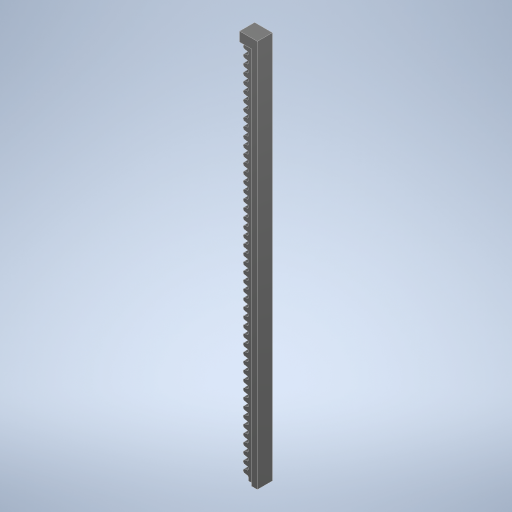
# Autodesk Inventor part: Hreben_Horizontal_cast
Saved by Autodesk Inventor 2024.2 (Build 282272000, 272)
## iProperties
Created: 2025-06-02
Part Number: Hreben_Horizontal_cast
Material: Termoplastická pryskyřice
Document SubType Name: Modeling
Designer: Elite
Density: 1.28 g/cm^3
Appearance: Hladká – černá
Mass: 4.51235 g
Surface Area: 29.4448 cm^2
Volume: 3.52528 cm^3
Author: Elite
Autodesk Inventor part; units mm, degrees
(part 1 of 2)
ref_plane "YZ Plane" through (0, 0, 0) normal (1, 0, 0) x (0, 1, 0)
ref_plane "XZ Plane" through (0, 0, 0) normal (0, 1, 0) x (-1, 0, 0)
ref_plane "XY Plane" through (0, 0, 0) normal (0, 0, 1) x (1, 0, 0)
sketch "Náčrt1" plane through (0, 0, 0) normal (0, 0, 1) x (1, 0, 0)
  line L0 (-2.539999, 6.35) -> (0, 6.35)
  line L1 (-2.539999, 6.35) -> (-3.809999, 5.08)
  line L2 (-3.809999, 5.08) -> (-5.079999, 5.08)
  line L3 (-5.079999, 5.08) -> (-5.079999, 1.27)
  line L4 (-5.079999, 1.27) -> (-3.809999, 1.27)
  line L5 (-3.809999, 1.27) -> (-2.539999, 0)
  line L6 (-2.539999, 0) -> (0, 0)
  line L7 (0, 0) -> (0, 6.35)
  constraints: 16 end point
extrude "Vysunutí1" add sketch "Náčrt1" against normal blind 160
sketch "Náčrt2" plane through (-3.809999, 5.08, 0) normal (0, 1, 0) x (1, 0, 0)
  line L0 (0, 0) -> (-1.27, 0)
  line L1 (0, 0) -> (0, 160)
  line L2 (-1.27, 160) -> (0, 160)
  line L3 (-1.27, 0) -> (-1.27, 160)
  arc A0 (-1.678461, 2.998415) -> (-1.27, 3.497336) centre (-1.778009, 3.496575) ccw
  arc A1 (-2.97646, 2.739034) -> (-3.389, 2.240304) centre (-2.881172, 2.240226) ccw
  arc A2 (-3.389, 1.845748) -> (-2.971901, 1.32351) centre (-2.881505, 1.82339) ccw
  line L4 (-2.990322, 1.327194) -> (-2.971901, 1.32351)
  arc A3 (-1.27, 0.566986) -> (-1.677758, 1.064456) centre (-1.777338, 0.566986) ccw
  line L5 (-1.27, 3.868884) -> (-1.27, 3.495814)
  line L6 (-1.27, 0) -> (-1.27, 160)
  line L7 (-2.971901, 1.32351) -> (-1.677758, 1.064456)
  line L8 (-3.389, 1.845748) -> (-3.389, 2.24059)
  line L9 (-2.97646, 2.739034) -> (-1.678461, 2.998415)
  line L10 (-1.27, 0.566986) -> (-1.27, 3.868884)
  arc A4 (-1.678461, 6.300312) -> (-1.27, 6.799234) centre (-1.778009, 6.798472) ccw
  arc A5 (-2.97646, 6.040931) -> (-3.389, 5.542202) centre (-2.881172, 5.542123) ccw
  arc A6 (-3.389, 5.147645) -> (-2.971901, 4.625407) centre (-2.881505, 5.125287) ccw
  line L11 (-2.990322, 4.629092) -> (-2.971901, 4.625407)
  arc A7 (-1.27, 3.868884) -> (-1.677758, 4.366353) centre (-1.777338, 3.868884) ccw
  line L12 (-1.27, 7.170781) -> (-1.27, 6.797711)
  line L13 (-2.971901, 4.625407) -> (-1.677758, 4.366353)
  line L14 (-3.389, 5.147645) -> (-3.389, 5.542488)
  line L15 (-2.97646, 6.040931) -> (-1.678461, 6.300312)
  line L16 (-1.27, 3.868884) -> (-1.27, 7.170781)
  arc A8 (-1.678461, 9.602209) -> (-1.27, 10.101131) centre (-1.778009, 10.10037) ccw
  arc A9 (-2.97646, 9.342828) -> (-3.389, 8.844099) centre (-2.881172, 8.844021) ccw
  arc A10 (-3.389, 8.449542) -> (-2.971901, 7.927305) centre (-2.881505, 8.427184) ccw
  line L17 (-2.990322, 7.930989) -> (-2.971901, 7.927305)
  arc A11 (-1.27, 7.170781) -> (-1.677758, 7.668251) centre (-1.777338, 7.170781) ccw
  line L18 (-1.27, 10.472678) -> (-1.27, 10.099608)
  line L19 (-2.971901, 7.927305) -> (-1.677758, 7.668251)
  line L20 (-3.389, 8.449542) -> (-3.389, 8.844385)
  line L21 (-2.97646, 9.342828) -> (-1.678461, 9.602209)
  line L22 (-1.27, 7.170781) -> (-1.27, 10.472678)
  arc A12 (-1.678461, 12.904106) -> (-1.27, 13.403028) centre (-1.778009, 13.402267) ccw
  arc A13 (-2.97646, 12.644726) -> (-3.389, 12.145996) centre (-2.881172, 12.145918) ccw
  arc A14 (-3.389, 11.751439) -> (-2.971901, 11.229202) centre (-2.881505, 11.729081) ccw
  line L23 (-2.990322, 11.232886) -> (-2.971901, 11.229202)
  arc A15 (-1.27, 10.472678) -> (-1.677758, 10.970148) centre (-1.777338, 10.472678) ccw
  line L24 (-1.27, 13.774575) -> (-1.27, 13.401505)
  line L25 (-2.971901, 11.229202) -> (-1.677758, 10.970148)
  line L26 (-3.389, 11.751439) -> (-3.389, 12.146282)
  line L27 (-2.97646, 12.644726) -> (-1.678461, 12.904106)
  line L28 (-1.27, 10.472678) -> (-1.27, 13.774575)
  arc A16 (-1.678461, 16.206003) -> (-1.27, 16.704925) centre (-1.778009, 16.704164) ccw
  arc A17 (-2.97646, 15.946623) -> (-3.389, 15.447893) centre (-2.881172, 15.447815) ccw
  arc A18 (-3.389, 15.053337) -> (-2.971901, 14.531099) centre (-2.881505, 15.030979) ccw
  line L29 (-2.990322, 14.534783) -> (-2.971901, 14.531099)
  arc A19 (-1.27, 13.774575) -> (-1.677758, 14.272045) centre (-1.777338, 13.774575) ccw
  line L30 (-1.27, 17.076472) -> (-1.27, 16.703403)
  line L31 (-2.971901, 14.531099) -> (-1.677758, 14.272045)
  line L32 (-3.389, 15.053337) -> (-3.389, 15.448179)
  line L33 (-2.97646, 15.946623) -> (-1.678461, 16.206003)
  line L34 (-1.27, 13.774575) -> (-1.27, 17.076472)
  arc A20 (-1.678461, 19.507901) -> (-1.27, 20.006822) centre (-1.778009, 20.006061) ccw
  arc A21 (-2.97646, 19.24852) -> (-3.389, 18.74979) centre (-2.881172, 18.749712) ccw
  arc A22 (-3.389, 18.355234) -> (-2.971901, 17.832996) centre (-2.881505, 18.332876) ccw
  line L35 (-2.990322, 17.83668) -> (-2.971901, 17.832996)
  arc A23 (-1.27, 17.076472) -> (-1.677758, 17.573942) centre (-1.777338, 17.076472) ccw
  line L36 (-1.27, 20.37837) -> (-1.27, 20.0053)
  line L37 (-2.971901, 17.832996) -> (-1.677758, 17.573942)
  line L38 (-3.389, 18.355234) -> (-3.389, 18.750076)
  line L39 (-2.97646, 19.24852) -> (-1.678461, 19.507901)
  line L40 (-1.27, 17.076472) -> (-1.27, 20.37837)
  arc A24 (-1.678461, 22.809798) -> (-1.27, 23.30872) centre (-1.778009, 23.307958) ccw
  arc A25 (-2.97646, 22.550417) -> (-3.389, 22.051688) centre (-2.881172, 22.051609) ccw
  arc A26 (-3.389, 21.657131) -> (-2.971901, 21.134893) centre (-2.881505, 21.634773) ccw
  line L41 (-2.990322, 21.138578) -> (-2.971901, 21.134893)
  arc A27 (-1.27, 20.37837) -> (-1.677758, 20.875839) centre (-1.777338, 20.37837) ccw
  line L42 (-1.27, 23.680267) -> (-1.27, 23.307197)
  line L43 (-2.971901, 21.134893) -> (-1.677758, 20.875839)
  line L44 (-3.389, 21.657131) -> (-3.389, 22.051974)
  line L45 (-2.97646, 22.550417) -> (-1.678461, 22.809798)
  line L46 (-1.27, 20.37837) -> (-1.27, 23.680267)
  arc A28 (-1.678461, 26.111695) -> (-1.27, 26.610617) centre (-1.778009, 26.609856) ccw
  arc A29 (-2.97646, 25.852314) -> (-3.389, 25.353585) centre (-2.881172, 25.353507) ccw
  arc A30 (-3.389, 24.959028) -> (-2.971901, 24.436791) centre (-2.881505, 24.93667) ccw
  line L47 (-2.990322, 24.440475) -> (-2.971901, 24.436791)
  arc A31 (-1.27, 23.680267) -> (-1.677758, 24.177737) centre (-1.777338, 23.680267) ccw
  line L48 (-1.27, 26.982164) -> (-1.27, 26.609094)
  line L49 (-2.971901, 24.436791) -> (-1.677758, 24.177737)
  line L50 (-3.389, 24.959028) -> (-3.389, 25.353871)
  line L51 (-2.97646, 25.852314) -> (-1.678461, 26.111695)
  line L52 (-1.27, 23.680267) -> (-1.27, 26.982164)
  line L53 (-2.971901, 27.738688) -> (-1.677758, 27.479634)
  line L54 (-2.97646, 29.154212) -> (-1.678461, 29.413592)
  line L55 (-2.990322, 27.742372) -> (-2.971901, 27.738688)
  arc A32 (-2.97646, 29.154212) -> (-3.389, 28.655482) centre (-2.881172, 28.655404) ccw
  line L56 (-3.389, 28.260925) -> (-3.389, 28.655768)
  arc A33 (-3.389, 28.260925) -> (-2.971901, 27.738688) centre (-2.881505, 28.238567) ccw
  arc A34 (-1.27, 26.982164) -> (-1.677758, 27.479634) centre (-1.777338, 26.982164) ccw
  arc A35 (-1.678461, 29.413592) -> (-1.27, 29.912514) centre (-1.778009, 29.911753) ccw
  line L57 (-1.27, 30.284061) -> (-1.27, 29.910991)
  line L58 (-1.27, 26.982164) -> (-1.27, 30.284061)
  line L59 (-2.971901, 31.040585) -> (-1.677758, 30.781531)
  line L60 (-2.97646, 32.456109) -> (-1.678461, 32.715489)
  line L61 (-2.990322, 31.044269) -> (-2.971901, 31.040585)
  arc A36 (-2.97646, 32.456109) -> (-3.389, 31.957379) centre (-2.881172, 31.957301) ccw
  line L62 (-3.389, 31.562823) -> (-3.389, 31.957665)
  arc A37 (-3.389, 31.562823) -> (-2.971901, 31.040585) centre (-2.881505, 31.540465) ccw
  arc A38 (-1.27, 30.284061) -> (-1.677758, 30.781531) centre (-1.777338, 30.284061) ccw
  arc A39 (-1.678461, 32.715489) -> (-1.27, 33.214411) centre (-1.778009, 33.21365) ccw
  line L63 (-1.27, 33.585958) -> (-1.27, 33.212889)
  line L64 (-1.27, 30.284061) -> (-1.27, 33.585958)
  line L65 (-2.971901, 34.342482) -> (-1.677758, 34.083428)
  line L66 (-2.97646, 35.758006) -> (-1.678461, 36.017387)
  line L67 (-2.990322, 34.346166) -> (-2.971901, 34.342482)
  arc A40 (-2.97646, 35.758006) -> (-3.389, 35.259276) centre (-2.881172, 35.259198) ccw
  line L68 (-3.389, 34.86472) -> (-3.389, 35.259562)
  arc A41 (-3.389, 34.86472) -> (-2.971901, 34.342482) centre (-2.881505, 34.842362) ccw
  arc A42 (-1.27, 33.585958) -> (-1.677758, 34.083428) centre (-1.777338, 33.585958) ccw
  arc A43 (-1.678461, 36.017387) -> (-1.27, 36.516308) centre (-1.778009, 36.515547) ccw
  line L69 (-1.27, 36.887856) -> (-1.27, 36.514786)
  line L70 (-1.27, 33.585958) -> (-1.27, 36.887856)
  line L71 (-2.971901, 37.644379) -> (-1.677758, 37.385325)
  line L72 (-2.97646, 39.059903) -> (-1.678461, 39.319284)
  line L73 (-2.990322, 37.648064) -> (-2.971901, 37.644379)
  arc A44 (-2.97646, 39.059903) -> (-3.389, 38.561174) centre (-2.881172, 38.561095) ccw
  line L74 (-3.389, 38.166617) -> (-3.389, 38.56146)
  arc A45 (-3.389, 38.166617) -> (-2.971901, 37.644379) centre (-2.881505, 38.144259) ccw
  arc A46 (-1.27, 36.887856) -> (-1.677758, 37.385325) centre (-1.777338, 36.887856) ccw
  arc A47 (-1.678461, 39.319284) -> (-1.27, 39.818206) centre (-1.778009, 39.817444) ccw
  line L75 (-1.27, 40.189753) -> (-1.27, 39.816683)
  line L76 (-1.27, 36.887856) -> (-1.27, 40.189753)
  line L77 (-2.971901, 40.946276) -> (-1.677758, 40.687223)
  line L78 (-2.97646, 42.3618) -> (-1.678461, 42.621181)
  line L79 (-2.990322, 40.949961) -> (-2.971901, 40.946276)
  arc A48 (-2.97646, 42.3618) -> (-3.389, 41.863071) centre (-2.881172, 41.862993) ccw
  line L80 (-3.389, 41.468514) -> (-3.389, 41.863357)
  arc A49 (-3.389, 41.468514) -> (-2.971901, 40.946276) centre (-2.881505, 41.446156) ccw
  arc A50 (-1.27, 40.189753) -> (-1.677758, 40.687223) centre (-1.777338, 40.189753) ccw
  arc A51 (-1.678461, 42.621181) -> (-1.27, 43.120103) centre (-1.778009, 43.119342) ccw
  line L81 (-1.27, 43.49165) -> (-1.27, 43.11858)
  line L82 (-1.27, 40.189753) -> (-1.27, 43.49165)
  line L83 (-2.971901, 44.248174) -> (-1.677758, 43.98912)
  line L84 (-2.97646, 45.663698) -> (-1.678461, 45.923078)
  line L85 (-2.990322, 44.251858) -> (-2.971901, 44.248174)
  arc A52 (-2.97646, 45.663698) -> (-3.389, 45.164968) centre (-2.881172, 45.16489) ccw
  line L86 (-3.389, 44.770411) -> (-3.389, 45.165254)
  arc A53 (-3.389, 44.770411) -> (-2.971901, 44.248174) centre (-2.881505, 44.748053) ccw
  arc A54 (-1.27, 43.49165) -> (-1.677758, 43.98912) centre (-1.777338, 43.49165) ccw
  arc A55 (-1.678461, 45.923078) -> (-1.27, 46.422) centre (-1.778009, 46.421239) ccw
  line L87 (-1.27, 46.793547) -> (-1.27, 46.420477)
  line L88 (-1.27, 43.49165) -> (-1.27, 46.793547)
  arc A56 (-1.678461, 49.224975) -> (-1.27, 49.723897) centre (-1.778009, 49.723136) ccw
  arc A57 (-2.97646, 48.965595) -> (-3.389, 48.466865) centre (-2.881172, 48.466787) ccw
  arc A58 (-3.389, 48.072309) -> (-2.971901, 47.550071) centre (-2.881505, 48.049951) ccw
  line L89 (-2.990322, 47.553755) -> (-2.971901, 47.550071)
  arc A59 (-1.27, 46.793547) -> (-1.677758, 47.291017) centre (-1.777338, 46.793547) ccw
  line L90 (-1.27, 50.095444) -> (-1.27, 49.722375)
  line L91 (-2.971901, 47.550071) -> (-1.677758, 47.291017)
  line L92 (-3.389, 48.072309) -> (-3.389, 48.467151)
  line L93 (-2.97646, 48.965595) -> (-1.678461, 49.224975)
  line L94 (-1.27, 46.793547) -> (-1.27, 50.095444)
  line L95 (-2.971901, 50.851968) -> (-1.677758, 50.592914)
  line L96 (-2.97646, 52.267492) -> (-1.678461, 52.526873)
  line L97 (-2.990322, 50.855652) -> (-2.971901, 50.851968)
  arc A60 (-2.97646, 52.267492) -> (-3.389, 51.768762) centre (-2.881172, 51.768684) ccw
  line L98 (-3.389, 51.374206) -> (-3.389, 51.769048)
  arc A61 (-3.389, 51.374206) -> (-2.971901, 50.851968) centre (-2.881505, 51.351848) ccw
  arc A62 (-1.27, 50.095444) -> (-1.677758, 50.592914) centre (-1.777338, 50.095444) ccw
  arc A63 (-1.678461, 52.526873) -> (-1.27, 53.025794) centre (-1.778009, 53.025033) ccw
  line L99 (-1.27, 53.397342) -> (-1.27, 53.024272)
  line L100 (-1.27, 50.095444) -> (-1.27, 53.397342)
  line L101 (-2.971901, 54.153865) -> (-1.677758, 53.894811)
  line L102 (-2.97646, 55.569389) -> (-1.678461, 55.82877)
  line L103 (-2.990322, 54.15755) -> (-2.971901, 54.153865)
  arc A64 (-2.97646, 55.569389) -> (-3.389, 55.07066) centre (-2.881172, 55.070581) ccw
  line L104 (-3.389, 54.676103) -> (-3.389, 55.070946)
  arc A65 (-3.389, 54.676103) -> (-2.971901, 54.153865) centre (-2.881505, 54.653745) ccw
  arc A66 (-1.27, 53.397342) -> (-1.677758, 53.894811) centre (-1.777338, 53.397342) ccw
  arc A67 (-1.678461, 55.82877) -> (-1.27, 56.327692) centre (-1.778009, 56.32693) ccw
  line L105 (-1.27, 56.699239) -> (-1.27, 56.326169)
  line L106 (-1.27, 53.397342) -> (-1.27, 56.699239)
  line L107 (-2.971901, 57.455762) -> (-1.677758, 57.196709)
  line L108 (-2.97646, 58.871286) -> (-1.678461, 59.130667)
  line L109 (-2.990322, 57.459447) -> (-2.971901, 57.455762)
  arc A68 (-2.97646, 58.871286) -> (-3.389, 58.372557) centre (-2.881172, 58.372479) ccw
  line L110 (-3.389, 57.978) -> (-3.389, 58.372843)
  arc A69 (-3.389, 57.978) -> (-2.971901, 57.455762) centre (-2.881505, 57.955642) ccw
  arc A70 (-1.27, 56.699239) -> (-1.677758, 57.196709) centre (-1.777338, 56.699239) ccw
  arc A71 (-1.678461, 59.130667) -> (-1.27, 59.629589) centre (-1.778009, 59.628828) ccw
  line L111 (-1.27, 60.001136) -> (-1.27, 59.628066)
  line L112 (-1.27, 56.699239) -> (-1.27, 60.001136)
  line L113 (-2.971901, 60.75766) -> (-1.677758, 60.498606)
  line L114 (-2.97646, 62.173184) -> (-1.678461, 62.432564)
  line L115 (-2.990322, 60.761344) -> (-2.971901, 60.75766)
  arc A72 (-2.97646, 62.173184) -> (-3.389, 61.674454) centre (-2.881172, 61.674376) ccw
  line L116 (-3.389, 61.279897) -> (-3.389, 61.67474)
  arc A73 (-3.389, 61.279897) -> (-2.971901, 60.75766) centre (-2.881505, 61.257539) ccw
  arc A74 (-1.27, 60.001136) -> (-1.677758, 60.498606) centre (-1.777338, 60.001136) ccw
  arc A75 (-1.678461, 62.432564) -> (-1.27, 62.931486) centre (-1.778009, 62.930725) ccw
  line L117 (-1.27, 63.303033) -> (-1.27, 62.929963)
  line L118 (-1.27, 60.001136) -> (-1.27, 63.303033)
  line L119 (-2.971901, 64.059557) -> (-1.677758, 63.800503)
  line L120 (-2.97646, 65.475081) -> (-1.678461, 65.734461)
  line L121 (-2.990322, 64.063241) -> (-2.971901, 64.059557)
  arc A76 (-2.97646, 65.475081) -> (-3.389, 64.976351) centre (-2.881172, 64.976273) ccw
  line L122 (-3.389, 64.581795) -> (-3.389, 64.976637)
  arc A77 (-3.389, 64.581795) -> (-2.971901, 64.059557) centre (-2.881505, 64.559437) ccw
  arc A78 (-1.27, 63.303033) -> (-1.677758, 63.800503) centre (-1.777338, 63.303033) ccw
  arc A79 (-1.678461, 65.734461) -> (-1.27, 66.233383) centre (-1.778009, 66.232622) ccw
  line L123 (-1.27, 66.60493) -> (-1.27, 66.231861)
  line L124 (-1.27, 63.303033) -> (-1.27, 66.60493)
  line L125 (-2.971901, 67.361454) -> (-1.677758, 67.1024)
  line L126 (-2.97646, 68.776978) -> (-1.678461, 69.036358)
  line L127 (-2.990322, 67.365138) -> (-2.971901, 67.361454)
  arc A80 (-2.97646, 68.776978) -> (-3.389, 68.278248) centre (-2.881172, 68.27817) ccw
  line L128 (-3.389, 67.883692) -> (-3.389, 68.278534)
  arc A81 (-3.389, 67.883692) -> (-2.971901, 67.361454) centre (-2.881505, 67.861334) ccw
  arc A82 (-1.27, 66.60493) -> (-1.677758, 67.1024) centre (-1.777338, 66.60493) ccw
  arc A83 (-1.678461, 69.036358) -> (-1.27, 69.53528) centre (-1.778009, 69.534519) ccw
  line L129 (-1.27, 69.906828) -> (-1.27, 69.533758)
  line L130 (-1.27, 66.60493) -> (-1.27, 69.906828)
  arc A84 (-1.678461, 72.338256) -> (-1.27, 72.837178) centre (-1.778009, 72.836416) ccw
  arc A85 (-2.97646, 72.078875) -> (-3.389, 71.580145) centre (-2.881172, 71.580067) ccw
  arc A86 (-3.389, 71.185589) -> (-2.971901, 70.663351) centre (-2.881505, 71.163231) ccw
  line L131 (-2.990322, 70.667035) -> (-2.971901, 70.663351)
  arc A87 (-1.27, 69.906828) -> (-1.677758, 70.404297) centre (-1.777338, 69.906828) ccw
  line L132 (-1.27, 73.208725) -> (-1.27, 72.835655)
  line L133 (-2.971901, 70.663351) -> (-1.677758, 70.404297)
  line L134 (-3.389, 71.185589) -> (-3.389, 71.580432)
  line L135 (-2.97646, 72.078875) -> (-1.678461, 72.338256)
  line L136 (-1.27, 69.906828) -> (-1.27, 73.208725)
  line L137 (-2.971901, 73.965248) -> (-1.677758, 73.706195)
  line L138 (-2.97646, 75.380772) -> (-1.678461, 75.640153)
  line L139 (-2.990322, 73.968933) -> (-2.971901, 73.965248)
  arc A88 (-2.97646, 75.380772) -> (-3.389, 74.882043) centre (-2.881172, 74.881965) ccw
  line L140 (-3.389, 74.487486) -> (-3.389, 74.882329)
  arc A89 (-3.389, 74.487486) -> (-2.971901, 73.965248) centre (-2.881505, 74.465128) ccw
  arc A90 (-1.27, 73.208725) -> (-1.677758, 73.706195) centre (-1.777338, 73.208725) ccw
  arc A91 (-1.678461, 75.640153) -> (-1.27, 76.139075) centre (-1.778009, 76.138314) ccw
  line L141 (-1.27, 76.510622) -> (-1.27, 76.137552)
  line L142 (-1.27, 73.208725) -> (-1.27, 76.510622)
  line L143 (-2.971901, 77.267146) -> (-1.677758, 77.008092)
  line L144 (-2.97646, 78.68267) -> (-1.678461, 78.94205)
  line L145 (-2.990322, 77.27083) -> (-2.971901, 77.267146)
  arc A92 (-2.97646, 78.68267) -> (-3.389, 78.18394) centre (-2.881172, 78.183862) ccw
  line L146 (-3.389, 77.789383) -> (-3.389, 78.184226)
  arc A93 (-3.389, 77.789383) -> (-2.971901, 77.267146) centre (-2.881505, 77.767025) ccw
  arc A94 (-1.27, 76.510622) -> (-1.677758, 77.008092) centre (-1.777338, 76.510622) ccw
  arc A95 (-1.678461, 78.94205) -> (-1.27, 79.440972) centre (-1.778009, 79.440211) ccw
  line L147 (-1.27, 79.812519) -> (-1.27, 79.439449)
  line L148 (-1.27, 76.510622) -> (-1.27, 79.812519)
  line L149 (-2.971901, 80.569043) -> (-1.677758, 80.309989)
  line L150 (-2.97646, 81.984567) -> (-1.678461, 82.243947)
  line L151 (-2.990322, 80.572727) -> (-2.971901, 80.569043)
  arc A96 (-2.97646, 81.984567) -> (-3.389, 81.485837) centre (-2.881172, 81.485759) ccw
  line L152 (-3.389, 81.091281) -> (-3.389, 81.486123)
  arc A97 (-3.389, 81.091281) -> (-2.971901, 80.569043) centre (-2.881505, 81.068923) ccw
  arc A98 (-1.27, 79.812519) -> (-1.677758, 80.309989) centre (-1.777338, 79.812519) ccw
  arc A99 (-1.678461, 82.243947) -> (-1.27, 82.742869) centre (-1.778009, 82.742108) ccw
  line L153 (-1.27, 83.114416) -> (-1.27, 82.741347)
  line L154 (-1.27, 79.812519) -> (-1.27, 83.114416)
  line L155 (-2.971901, 83.87094) -> (-1.677758, 83.611886)
  line L156 (-2.97646, 85.286464) -> (-1.678461, 85.545844)
  line L157 (-2.990322, 83.874624) -> (-2.971901, 83.87094)
  arc A100 (-2.97646, 85.286464) -> (-3.389, 84.787734) centre (-2.881172, 84.787656) ccw
  line L158 (-3.389, 84.393178) -> (-3.389, 84.78802)
  arc A101 (-3.389, 84.393178) -> (-2.971901, 83.87094) centre (-2.881505, 84.37082) ccw
  arc A102 (-1.27, 83.114416) -> (-1.677758, 83.611886) centre (-1.777338, 83.114416) ccw
  arc A103 (-1.678461, 85.545844) -> (-1.27, 86.044766) centre (-1.778009, 86.044005) ccw
  line L159 (-1.27, 86.416314) -> (-1.27, 86.043244)
  line L160 (-1.27, 83.114416) -> (-1.27, 86.416314)
  line L161 (-2.971901, 87.172837) -> (-1.677758, 86.913783)
  line L162 (-2.97646, 88.588361) -> (-1.678461, 88.847742)
  line L163 (-2.990322, 87.176521) -> (-2.971901, 87.172837)
  arc A104 (-2.97646, 88.588361) -> (-3.389, 88.089631) centre (-2.881172, 88.089553) ccw
  line L164 (-3.389, 87.695075) -> (-3.389, 88.089918)
  arc A105 (-3.389, 87.695075) -> (-2.971901, 87.172837) centre (-2.881505, 87.672717) ccw
  arc A106 (-1.27, 86.416314) -> (-1.677758, 86.913783) centre (-1.777338, 86.416314) ccw
  arc A107 (-1.678461, 88.847742) -> (-1.27, 89.346664) centre (-1.778009, 89.345902) ccw
  line L165 (-1.27, 89.718211) -> (-1.27, 89.345141)
  line L166 (-1.27, 86.416314) -> (-1.27, 89.718211)
  arc A108 (-1.27, 89.718211) -> (-1.677758, 90.215681) centre (-1.777338, 89.718211) ccw
  line L167 (-2.971901, 90.474734) -> (-1.677758, 90.215681)
  line L168 (-2.990322, 90.478419) -> (-2.971901, 90.474734)
  arc A109 (-3.389, 90.996972) -> (-2.971901, 90.474734) centre (-2.881505, 90.974614) ccw
  arc A110 (-2.97646, 91.890258) -> (-3.389, 91.391529) centre (-2.881172, 91.391451) ccw
  line L169 (-2.97646, 91.890258) -> (-1.678461, 92.149639)
  line L170 (-1.27, 89.718211) -> (-1.27, 93.020108)
  arc A111 (-1.678461, 92.149639) -> (-1.27, 92.648561) centre (-1.778009, 92.647799) ccw
  line L171 (-1.27, 93.020108) -> (-1.27, 92.647038)
  line L172 (-3.389, 90.996972) -> (-3.389, 91.391815)
  arc A112 (-1.27, 93.020108) -> (-1.677758, 93.517578) centre (-1.777338, 93.020108) ccw
  line L173 (-2.971901, 93.776632) -> (-1.677758, 93.517578)
  line L174 (-2.990322, 93.780316) -> (-2.971901, 93.776632)
  arc A113 (-3.389, 94.298869) -> (-2.971901, 93.776632) centre (-2.881505, 94.276511) ccw
  line L175 (-3.389, 94.298869) -> (-3.389, 94.693712)
  arc A114 (-2.97646, 95.192156) -> (-3.389, 94.693426) centre (-2.881172, 94.693348) ccw
  line L176 (-1.27, 93.020108) -> (-1.27, 96.322005)
  line L177 (-2.97646, 95.192156) -> (-1.678461, 95.451536)
  arc A115 (-1.678461, 95.451536) -> (-1.27, 95.950458) centre (-1.778009, 95.949697) ccw
  line L178 (-1.27, 96.322005) -> (-1.27, 95.948935)
  arc A116 (-1.678461, 98.753433) -> (-1.27, 99.252355) centre (-1.778009, 99.251594) ccw
  arc A117 (-1.27, 99.623902) -> (-1.677758, 100.121372) centre (-1.777338, 99.623902) ccw
  line L179 (-1.27, 99.623902) -> (-1.27, 99.250833)
  arc A118 (-2.97646, 98.494053) -> (-3.389, 97.995323) centre (-2.881172, 97.995245) ccw
  line L180 (-2.990322, 97.082213) -> (-2.971901, 97.078529)
  arc A119 (-3.389, 97.600767) -> (-2.971901, 97.078529) centre (-2.881505, 97.578409) ccw
  line L181 (-2.971901, 100.380426) -> (-1.677758, 100.121372)
  line L182 (-2.990322, 100.38411) -> (-2.971901, 100.380426)
  arc A120 (-3.389, 100.902664) -> (-2.971901, 100.380426) centre (-2.881505, 100.880306) ccw
  line L183 (-3.389, 100.902664) -> (-3.389, 101.297506)
  arc A121 (-2.97646, 101.79595) -> (-3.389, 101.29722) centre (-2.881172, 101.297142) ccw
  line L184 (-2.97646, 101.79595) -> (-1.678461, 102.05533)
  line L185 (-1.27, 99.623902) -> (-1.27, 102.925799)
  arc A122 (-1.678461, 102.05533) -> (-1.27, 102.554252) centre (-1.778009, 102.553491) ccw
  line L186 (-1.27, 102.925799) -> (-1.27, 102.55273)
  arc A123 (-1.27, 96.322005) -> (-1.677758, 96.819475) centre (-1.777338, 96.322005) ccw
  line L187 (-2.971901, 97.078529) -> (-1.677758, 96.819475)
  line L188 (-2.97646, 98.494053) -> (-1.678461, 98.753433)
  line L189 (-3.389, 97.600767) -> (-3.389, 97.995609)
  line L190 (-1.27, 96.322005) -> (-1.27, 99.623902)
  arc A124 (-1.27, 102.925799) -> (-1.677758, 103.423269) centre (-1.777338, 102.925799) ccw
  line L191 (-2.971901, 103.682323) -> (-1.677758, 103.423269)
  line L192 (-2.990322, 103.686007) -> (-2.971901, 103.682323)
  arc A125 (-3.389, 104.204561) -> (-2.971901, 103.682323) centre (-2.881505, 104.182203) ccw
  line L193 (-3.389, 104.204561) -> (-3.389, 104.599404)
  arc A126 (-2.97646, 105.097847) -> (-3.389, 104.599117) centre (-2.881172, 104.599039) ccw
  line L194 (-2.97646, 105.097847) -> (-1.678461, 105.357228)
  line L195 (-1.27, 102.925799) -> (-1.27, 106.227697)
  arc A127 (-1.678461, 105.357228) -> (-1.27, 105.85615) centre (-1.778009, 105.855388) ccw
  line L196 (-1.27, 106.227697) -> (-1.27, 105.854627)
  arc A128 (-1.27, 106.227697) -> (-1.677758, 106.725166) centre (-1.777338, 106.227697) ccw
  line L197 (-2.971901, 106.98422) -> (-1.677758, 106.725166)
  line L198 (-2.990322, 106.987905) -> (-2.971901, 106.98422)
  arc A129 (-3.389, 107.506458) -> (-2.971901, 106.98422) centre (-2.881505, 107.4841) ccw
  line L199 (-3.389, 107.506458) -> (-3.389, 107.901301)
  arc A130 (-2.97646, 108.399744) -> (-3.389, 107.901015) centre (-2.881172, 107.900937) ccw
  line L200 (-2.97646, 108.399744) -> (-1.678461, 108.659125)
  line L201 (-1.27, 106.227697) -> (-1.27, 109.529594)
  arc A131 (-1.678461, 108.659125) -> (-1.27, 109.158047) centre (-1.778009, 109.157285) ccw
  line L202 (-1.27, 109.529594) -> (-1.27, 109.156524)
  arc A132 (-1.27, 109.529594) -> (-1.677758, 110.027064) centre (-1.777338, 109.529594) ccw
  line L203 (-2.971901, 110.286118) -> (-1.677758, 110.027064)
  line L204 (-2.990322, 110.289802) -> (-2.971901, 110.286118)
  line L205 (-3.389, 110.808355) -> (-3.389, 111.203198)
  arc A133 (-2.97646, 111.701641) -> (-3.389, 111.202912) centre (-2.881172, 111.202834) ccw
  line L206 (-2.97646, 111.701641) -> (-1.678461, 111.961022)
  arc A134 (-1.678461, 111.961022) -> (-1.27, 112.459944) centre (-1.778009, 112.459183) ccw
  line L207 (-1.27, 109.529594) -> (-1.27, 112.831491)
  line L208 (-1.27, 112.831491) -> (-1.27, 112.458421)
  arc A135 (-3.389, 110.808355) -> (-2.971901, 110.286118) centre (-2.881505, 110.785997) ccw
  arc A136 (-1.27, 112.831491) -> (-1.677758, 113.328961) centre (-1.777338, 112.831491) ccw
  line L209 (-2.971901, 113.588015) -> (-1.677758, 113.328961)
  line L210 (-2.990322, 113.591699) -> (-2.971901, 113.588015)
  arc A137 (-3.389, 114.110253) -> (-2.971901, 113.588015) centre (-2.881505, 114.087895) ccw
  arc A138 (-2.97646, 115.003539) -> (-3.389, 114.504809) centre (-2.881172, 114.504731) ccw
  line L211 (-2.97646, 115.003539) -> (-1.678461, 115.262919)
  line L212 (-1.27, 112.831491) -> (-1.27, 116.133388)
  arc A139 (-1.678461, 115.262919) -> (-1.27, 115.761841) centre (-1.778009, 115.76108) ccw
  line L213 (-1.27, 116.133388) -> (-1.27, 115.760319)
  line L214 (-3.389, 114.110253) -> (-3.389, 114.505095)
  arc A140 (-1.27, 116.133388) -> (-1.677758, 116.630858) centre (-1.777338, 116.133388) ccw
  line L215 (-2.971901, 116.889912) -> (-1.677758, 116.630858)
  line L216 (-2.990322, 116.893596) -> (-2.971901, 116.889912)
  arc A141 (-3.389, 117.41215) -> (-2.971901, 116.889912) centre (-2.881505, 117.389792) ccw
  line L217 (-3.389, 117.41215) -> (-3.389, 117.806992)
  arc A142 (-2.97646, 118.305436) -> (-3.389, 117.806706) centre (-2.881172, 117.806628) ccw
  line L218 (-1.27, 116.133388) -> (-1.27, 119.435285)
  line L219 (-2.97646, 118.305436) -> (-1.678461, 118.564816)
  arc A143 (-1.678461, 118.564816) -> (-1.27, 119.063738) centre (-1.778009, 119.062977) ccw
  line L220 (-1.27, 119.435285) -> (-1.27, 119.062216)
  arc A144 (-1.678461, 121.866714) -> (-1.27, 122.365636) centre (-1.778009, 122.364874) ccw
  arc A145 (-1.27, 122.737183) -> (-1.677758, 123.234652) centre (-1.777338, 122.737183) ccw
  line L221 (-1.27, 122.737183) -> (-1.27, 122.364113)
  arc A146 (-2.97646, 121.607333) -> (-3.389, 121.108603) centre (-2.881172, 121.108525) ccw
  line L222 (-2.990322, 120.195493) -> (-2.971901, 120.191809)
  arc A147 (-3.389, 120.714047) -> (-2.971901, 120.191809) centre (-2.881505, 120.691689) ccw
  line L223 (-2.971901, 123.493706) -> (-1.677758, 123.234652)
  line L224 (-2.990322, 123.497391) -> (-2.971901, 123.493706)
  arc A148 (-3.389, 124.015944) -> (-2.971901, 123.493706) centre (-2.881505, 123.993586) ccw
  line L225 (-3.389, 124.015944) -> (-3.389, 124.410787)
  arc A149 (-2.97646, 124.90923) -> (-3.389, 124.410501) centre (-2.881172, 124.410423) ccw
  line L226 (-2.97646, 124.90923) -> (-1.678461, 125.168611)
  line L227 (-1.27, 122.737183) -> (-1.27, 126.03908)
  arc A150 (-1.678461, 125.168611) -> (-1.27, 125.667533) centre (-1.778009, 125.666771) ccw
  line L228 (-1.27, 126.03908) -> (-1.27, 125.66601)
  arc A151 (-1.27, 119.435285) -> (-1.677758, 119.932755) centre (-1.777338, 119.435285) ccw
  line L229 (-2.971901, 120.191809) -> (-1.677758, 119.932755)
  line L230 (-2.97646, 121.607333) -> (-1.678461, 121.866714)
  line L231 (-3.389, 120.714047) -> (-3.389, 121.10889)
  line L232 (-1.27, 119.435285) -> (-1.27, 122.737183)
  arc A152 (-1.27, 126.03908) -> (-1.677758, 126.53655) centre (-1.777338, 126.03908) ccw
  line L233 (-2.971901, 126.795604) -> (-1.677758, 126.53655)
  line L234 (-2.990322, 126.799288) -> (-2.971901, 126.795604)
  arc A153 (-3.389, 127.317841) -> (-2.971901, 126.795604) centre (-2.881505, 127.295483) ccw
  line L235 (-3.389, 127.317841) -> (-3.389, 127.712684)
  arc A154 (-2.97646, 128.211127) -> (-3.389, 127.712398) centre (-2.881172, 127.71232) ccw
  line L236 (-2.97646, 128.211127) -> (-1.678461, 128.470508)
  line L237 (-1.27, 126.03908) -> (-1.27, 129.340977)
  arc A155 (-1.678461, 128.470508) -> (-1.27, 128.96943) centre (-1.778009, 128.968669) ccw
  line L238 (-1.27, 129.340977) -> (-1.27, 128.967907)
  arc A156 (-1.27, 129.340977) -> (-1.677758, 129.838447) centre (-1.777338, 129.340977) ccw
  line L239 (-2.971901, 130.097501) -> (-1.677758, 129.838447)
  line L240 (-2.990322, 130.101185) -> (-2.971901, 130.097501)
  arc A157 (-3.389, 130.619739) -> (-2.971901, 130.097501) centre (-2.881505, 130.59738) ccw
  line L241 (-3.389, 130.619739) -> (-3.389, 131.014581)
  arc A158 (-2.97646, 131.513025) -> (-3.389, 131.014295) centre (-2.881172, 131.014217) ccw
  line L242 (-2.97646, 131.513025) -> (-1.678461, 131.772405)
  line L243 (-1.27, 129.340977) -> (-1.27, 132.642874)
  arc A159 (-1.678461, 131.772405) -> (-1.27, 132.271327) centre (-1.778009, 132.270566) ccw
  line L244 (-1.27, 132.642874) -> (-1.27, 132.269805)
  arc A160 (-1.27, 132.642874) -> (-1.677758, 133.140344) centre (-1.777338, 132.642874) ccw
  line L245 (-2.971901, 133.399398) -> (-1.677758, 133.140344)
  line L246 (-2.990322, 133.403082) -> (-2.971901, 133.399398)
  line L247 (-3.389, 133.921636) -> (-3.389, 134.316478)
  arc A161 (-2.97646, 134.814922) -> (-3.389, 134.316192) centre (-2.881172, 134.316114) ccw
  line L248 (-2.97646, 134.814922) -> (-1.678461, 135.074302)
  arc A162 (-1.678461, 135.074302) -> (-1.27, 135.573224) centre (-1.778009, 135.572463) ccw
  line L249 (-1.27, 132.642874) -> (-1.27, 135.944771)
  line L250 (-1.27, 135.944771) -> (-1.27, 135.571702)
  arc A163 (-3.389, 133.921636) -> (-2.971901, 133.399398) centre (-2.881505, 133.899278) ccw
  arc A164 (-1.27, 135.944771) -> (-1.677758, 136.442241) centre (-1.777338, 135.944771) ccw
  line L251 (-2.971901, 136.701295) -> (-1.677758, 136.442241)
  line L252 (-2.990322, 136.704979) -> (-2.971901, 136.701295)
  arc A165 (-3.389, 137.223533) -> (-2.971901, 136.701295) centre (-2.881505, 137.201175) ccw
  arc A166 (-2.97646, 138.116819) -> (-3.389, 137.618089) centre (-2.881172, 137.618011) ccw
  line L253 (-2.97646, 138.116819) -> (-1.678461, 138.3762)
  line L254 (-1.27, 135.944771) -> (-1.27, 139.246669)
  arc A167 (-1.678461, 138.3762) -> (-1.27, 138.875122) centre (-1.778009, 138.87436) ccw
  line L255 (-1.27, 139.246669) -> (-1.27, 138.873599)
  line L256 (-3.389, 137.223533) -> (-3.389, 137.618376)
  arc A168 (-1.27, 139.246669) -> (-1.677758, 139.744138) centre (-1.777338, 139.246669) ccw
  line L257 (-2.971901, 140.003192) -> (-1.677758, 139.744138)
  line L258 (-2.990322, 140.006877) -> (-2.971901, 140.003192)
  arc A169 (-3.389, 140.52543) -> (-2.971901, 140.003192) centre (-2.881505, 140.503072) ccw
  arc A170 (-2.97646, 141.418716) -> (-3.389, 140.919987) centre (-2.881172, 140.919909) ccw
  line L259 (-2.97646, 141.418716) -> (-1.678461, 141.678097)
  line L260 (-1.27, 139.246669) -> (-1.27, 142.548566)
  arc A171 (-1.678461, 141.678097) -> (-1.27, 142.177019) centre (-1.778009, 142.176257) ccw
  line L261 (-1.27, 142.548566) -> (-1.27, 142.175496)
  line L262 (-3.389, 140.52543) -> (-3.389, 140.920273)
  arc A172 (-1.27, 142.548566) -> (-1.677758, 143.046036) centre (-1.777338, 142.548566) ccw
  line L263 (-2.971901, 143.30509) -> (-1.677758, 143.046036)
  line L264 (-2.990322, 143.308774) -> (-2.971901, 143.30509)
  arc A173 (-3.389, 143.827327) -> (-2.971901, 143.30509) centre (-2.881505, 143.804969) ccw
  line L265 (-3.389, 143.827327) -> (-3.389, 144.22217)
  arc A174 (-2.97646, 144.720613) -> (-3.389, 144.221884) centre (-2.881172, 144.221806) ccw
  line L266 (-1.27, 142.548566) -> (-1.27, 145.850463)
  line L267 (-2.97646, 144.720613) -> (-1.678461, 144.979994)
  arc A175 (-1.678461, 144.979994) -> (-1.27, 145.478916) centre (-1.778009, 145.478155) ccw
  line L268 (-1.27, 145.850463) -> (-1.27, 145.477393)
  arc A176 (-1.678461, 148.281891) -> (-1.27, 148.780813) centre (-1.778009, 148.780052) ccw
  arc A177 (-1.27, 149.15236) -> (-1.677758, 149.64983) centre (-1.777338, 149.15236) ccw
  line L269 (-1.27, 149.15236) -> (-1.27, 148.779291)
  arc A178 (-2.97646, 148.022511) -> (-3.389, 147.523781) centre (-2.881172, 147.523703) ccw
  line L270 (-2.990322, 146.610671) -> (-2.971901, 146.606987)
  arc A179 (-3.389, 147.129224) -> (-2.971901, 146.606987) centre (-2.881505, 147.106866) ccw
  line L271 (-2.971901, 149.908884) -> (-1.677758, 149.64983)
  line L272 (-2.990322, 149.912568) -> (-2.971901, 149.908884)
  arc A180 (-3.389, 150.431122) -> (-2.971901, 149.908884) centre (-2.881505, 150.408764) ccw
  line L273 (-3.389, 150.431122) -> (-3.389, 150.825964)
  arc A181 (-2.97646, 151.324408) -> (-3.389, 150.825678) centre (-2.881172, 150.8256) ccw
  line L274 (-2.97646, 151.324408) -> (-1.678461, 151.583788)
  line L275 (-1.27, 149.15236) -> (-1.27, 152.454257)
  arc A182 (-1.678461, 151.583788) -> (-1.27, 152.08271) centre (-1.778009, 152.081949) ccw
  line L276 (-1.27, 152.454257) -> (-1.27, 152.081188)
  arc A183 (-1.27, 145.850463) -> (-1.677758, 146.347933) centre (-1.777338, 145.850463) ccw
  line L277 (-2.971901, 146.606987) -> (-1.677758, 146.347933)
  line L278 (-2.97646, 148.022511) -> (-1.678461, 148.281891)
  line L279 (-3.389, 147.129224) -> (-3.389, 147.524067)
  line L280 (-1.27, 145.850463) -> (-1.27, 149.15236)
  arc A184 (-1.27, 152.454257) -> (-1.677758, 152.951727) centre (-1.777338, 152.454257) ccw
  line L281 (-2.971901, 153.210781) -> (-1.677758, 152.951727)
  line L282 (-2.990322, 153.214465) -> (-2.971901, 153.210781)
  arc A185 (-3.389, 153.733019) -> (-2.971901, 153.210781) centre (-2.881505, 153.710661) ccw
  line L283 (-3.389, 153.733019) -> (-3.389, 154.127862)
  arc A186 (-2.97646, 154.626305) -> (-3.389, 154.127575) centre (-2.881172, 154.127497) ccw
  line L284 (-2.97646, 154.626305) -> (-1.678461, 154.885686)
  line L285 (-1.27, 152.454257) -> (-1.27, 155.756155)
  arc A187 (-1.678461, 154.885686) -> (-1.27, 155.384608) centre (-1.778009, 155.383846) ccw
  line L286 (-1.27, 155.756155) -> (-1.27, 155.383085)
  arc A188 (-1.27, 155.756155) -> (-1.677758, 156.253624) centre (-1.777338, 155.756155) ccw
  line L287 (-2.971901, 156.512678) -> (-1.677758, 156.253624)
  line L288 (-2.990322, 156.516363) -> (-2.971901, 156.512678)
  arc A189 (-3.389, 157.034916) -> (-2.971901, 156.512678) centre (-2.881505, 157.012558) ccw
  line L289 (-3.389, 157.034916) -> (-3.389, 157.429759)
  arc A190 (-2.97646, 157.928202) -> (-3.389, 157.429473) centre (-2.881172, 157.429395) ccw
  line L290 (-2.97646, 157.928202) -> (-1.678461, 158.187583)
  line L291 (-1.27, 155.756155) -> (-1.27, 159.058052)
  arc A191 (-1.678461, 158.187583) -> (-1.27, 158.686505) centre (-1.778009, 158.685743) ccw
  line L292 (-1.27, 159.058052) -> (-1.27, 158.684982)
  point P0 (3.809999, 0)
  point P1 (-1.27, 3.410473)
  point P2 (-3.389, 2.240304)
  point P3 (-1.27, 6.71237)
  point P4 (-1.27, 10.014267)
  point P5 (-1.27, 13.316164)
  point P6 (-1.27, 16.618062)
  point P7 (-1.27, 19.919959)
  point P8 (-1.27, 23.221856)
  point P9 (-1.27, 26.523753)
  point P10 (-1.27, 29.82565)
  point P11 (-1.27, 33.127548)
  point P12 (-1.27, 36.429445)
  point P13 (-1.27, 39.731342)
  point P14 (-1.27, 43.033239)
  point P15 (-1.27, 46.335136)
  point P16 (-1.27, 49.637034)
  point P17 (-1.27, 52.938931)
  point P18 (-1.27, 56.240828)
  point P19 (-1.27, 59.542725)
  point P20 (-1.27, 62.844622)
  point P21 (-1.27, 66.14652)
  point P22 (-1.27, 69.448417)
  point P23 (-1.27, 72.750314)
  point P24 (-1.27, 76.052211)
  point P25 (-1.27, 79.354108)
  point P26 (-1.27, 82.656006)
  point P27 (-1.27, 85.957903)
  point P28 (-1.27, 89.2598)
  point P29 (-3.389, 88.089631)
  point P30 (-3.389, 71.580145)
  point P31 (-3.389, 64.976351)
  point P32 (-3.389, 41.863071)
  point P33 (-1.27, 29.912514)
  point P34 (-3.389, 25.353585)
  point P35 (-3.389, 22.051688)
  point P36 (-3.389, 18.74979)
  point P37 (-3.389, 15.447893)
  point P38 (-3.389, 12.145996)
  point P39 (-3.389, 8.844099)
  point P40 (-3.389, 5.542202)
  point P41 (-1.27, 92.561697)
  point P42 (-1.27, 95.863594)
  point P43 (-1.27, 99.165492)
  point P44 (-1.27, 102.467389)
  point P45 (-1.27, 105.769286)
  point P46 (-1.27, 109.071183)
  point P47 (-1.27, 112.37308)
  point P48 (-1.27, 115.674978)
  point P49 (-1.27, 118.976875)
  point P50 (-1.27, 122.278772)
  point P51 (-1.27, 125.580669)
  point P52 (-1.27, 128.882566)
  point P53 (-1.27, 132.184464)
  point P54 (-1.27, 135.486361)
  point P55 (-1.27, 138.788258)
  point P56 (-1.27, 139.246669)
  point P57 (-1.27, 142.090155)
  point P58 (-1.27, 145.392052)
  point P59 (-1.27, 148.693949)
  point P60 (-1.27, 151.995847)
  point P61 (-1.27, 155.297744)
  point P62 (-1.27, 158.599641)
  point P63 (-3.389, 117.806706)
  constraints: 624 end point, 480 point on circle, 192 centre point, 192 tangent, 50 point on line, 48 collinear